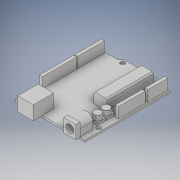
# Autodesk Inventor part: arduinoUno
Saved by Autodesk Inventor 2018 (Build 220112000, 112)
## iProperties
Created: 2020-03-26
Part Number: arduinoUno
Material: Generic
Document SubType Name: Modeling
Designer: natha
Density: 1 g/cm^3
Appearance: Default
Author: natha
Autodesk Inventor part; units mm, degrees
ref_plane "YZ Plane" through (0, 0, 0) normal (1, 0, 0) x (0, 1, 0)
ref_plane "XZ Plane" through (0, 0, 0) normal (0, 1, 0) x (-1, 0, 0)
ref_plane "XY Plane" through (0, 0, 0) normal (0, 0, 1) x (1, 0, 0)
sketch "Sketch1" plane through (0, 0, 0) normal (0, 1, 0) x (-1, 0, 0)
  line L0 (0, 0) -> (53.4, 0)
  line L1 (5, -68.6) -> (2.3639, -65.9639)
  line L2 (5, -68.6) -> (8.728, -68.6) construction
  line L3 (2.3639, -65.9639) -> (0.3639, -65.9639)
  line L4 (0.3639, -65.9639) -> (0, -65.6)
  line L5 (52.7794, -66.2206) -> (53.4, -65.6)
  line L6 (52.7794, -66.2206) -> (40.7794, -66.2206)
  line L7 (40.7794, -66.2206) -> (37.9652, -68.6)
  line L8 (37.9652, -68.6) -> (5, -68.6)
  line L9 (53.4, -65.6) -> (53.4, 0)
  line L10 (0, 0) -> (0, -65.6)
  circle A0 centre (36.6794, -65.9103) radius 1.7
  circle A1 centre (6.3639, -65.6) radius 1.7
  dimension "d2" = 135
  dimension "d3" = 135
  dimension "d10" = 12
  dimension "d12" = 135
  dimension "d13" = 3.4
  dimension "d14" = 3.4
  dimension "d15" = 4.1
  dimension "d16" = 4
  constraints: 22 end point, 5 horizontal, 2 centre point, 1 equal length, 1 perpendicular, 1 vertical
  measures "d2" angle of L2 L1
  measures "d3" angle of L3 L4
  measures "d10" distance of L5.start L6.end
  measures "d12" angle of L6 L5
  measures "d13" diameter of A0
  measures "d14" diameter of A1
  measures "d15" horizontal distance of A0.centre L6.end
  measures "d16" horizontal distance of L1.end A1.centre
extrude "Extrusion1" add sketch "Sketch1" along normal blind 1.5
sketch "Sketch2" plane through (0, 1.5, 0) normal (0, 1, 0) x (1, 0, 0)
  circle A0 centre (-50.9, 14.75) radius 1.7
  line L0 (-53.4, 0) -> (0, 0) projected
  line L1 (-53.4, 65.6) -> (-53.4, 0) projected
  circle A1 centre (-2.5, 13.4) radius 1.7
  line L2 (0, 0) -> (0, 65.6) projected
  dimension "d19" = 3.4
  dimension "d20" = 14.75
  dimension "d21" = 2.5
  dimension "d22" = 3.4
  dimension "d23" = 13.4
  dimension "d24" = 2.5
  constraints: 2 centre point
  measures "d19" diameter of A0
  measures "d20" distance from line of L0 A0.centre
  measures "d21" distance from line of L1 A0.centre
  measures "d22" diameter of A1
  measures "d23" distance from line of L0 A1.centre
  measures "d24" distance from line of L2 A1.centre
extrude "Extrusion2" cut sketch "Sketch2" against normal blind 1.5
sketch "Sketch3" plane through (0, 1.5, 0) normal (0, 1, 0) x (1, 0, 0)
  line L0 (-1, 64.9639) -> (-3.3, 64.9639)
  line L1 (-3.3, 64.9639) -> (-3.3, 49.4639)
  line L2 (-3.3, 49.4639) -> (-1, 49.4639)
  line L3 (-1, 49.4639) -> (-1, 64.9639)
  line L4 (-0.3639, 65.9639) -> (-2.3639, 65.9639) projected
  line L5 (0, 0) -> (0, 65.6) projected
  line L6 (-3.3, 47.4639) -> (-1, 47.4639)
  line L7 (-1, 47.4639) -> (-1, 26.9639)
  line L8 (-1, 26.9639) -> (-3.3, 26.9639)
  line L9 (-3.3, 26.9639) -> (-3.3, 47.4639)
  line L10 (-52.4, 44.7206) -> (-50.1, 44.7206)
  line L11 (-50.1, 44.7206) -> (-50.1, 65.2206)
  line L12 (-50.1, 65.2206) -> (-52.4, 65.2206)
  line L13 (-52.4, 65.2206) -> (-52.4, 44.7206)
  line L14 (-53.4, 65.6) -> (-53.4, 0) projected
  line L15 (-40.7794, 66.2206) -> (-52.7794, 66.2206) projected
  line L16 (-52.4, 43.7206) -> (-50.1, 43.7206)
  line L17 (-50.1, 43.7206) -> (-50.1, 17.6206)
  line L18 (-50.1, 17.6206) -> (-52.4, 17.6206)
  line L19 (-52.4, 17.6206) -> (-52.4, 43.7206)
  dimension "d27" = 1
  dimension "d28" = 15.5
  dimension "d29" = 2.3
  dimension "d30" = 1
  dimension "d31" = 2
  dimension "d32" = 2.3
  dimension "d33" = 20.5
  dimension "d34" = 1
  dimension "d35" = 1
  dimension "d36" = 2.3
  dimension "d37" = 20.5
  dimension "d38" = 26.1
  dimension "d39" = 1
  constraints: 32 end point, 8 parallel, 4 horizontal, 4 perpendicular
  measures "d27" distance between parallel lines of L4 L0
  measures "d28" distance between parallel lines of L2 L0
  measures "d29" distance between parallel lines of L3 L1
  measures "d30" distance between parallel lines of L3 L5
  measures "d31" distance between parallel lines of L2 L6
  measures "d32" distance between parallel lines of L9 L7
  measures "d33" distance between parallel lines of L8 L6
  measures "d34" distance between parallel lines of L14 L13
  measures "d35" distance between parallel lines of L15 L12
  measures "d36" distance between parallel lines of L13 L11
  measures "d37" distance between parallel lines of L10 L12
  measures "d38" distance of L16.end L17.end
  measures "d39" distance between parallel lines of L10 L16
extrude "Extrusion3" add sketch "Sketch3" along normal blind 8.3
sketch "Sketch4" plane through (0, 1.5, 0) normal (0, 1, 0) x (1, 0, 0)
  line L0 (-20.8, 27.85) -> (-10.8, 27.85)
  line L1 (-10.8, 27.85) -> (-10.8, 63.6)
  line L2 (-10.8, 63.6) -> (-20.8, 63.6)
  line L3 (-20.8, 63.6) -> (-20.8, 27.85)
  line L4 (-3.3, 47.4639) -> (-3.3, 26.9639) projected
  line L5 (-5, 68.6) -> (-37.9652, 68.6) projected
  point P0 (0, 0)
  dimension "d42" = 10
  dimension "d43" = 35.75
  dimension "d44" = 7.5
  dimension "d45" = 5
  constraints: 8 end point, 2 parallel, 1 horizontal, 1 perpendicular
  measures "d42" distance of L2.end L1.end
  measures "d43" distance of L1.end L0.end
  measures "d44" distance between parallel lines of L1 L4
  measures "d45" distance between parallel lines of L5 L2
extrude "Extrusion4" add sketch "Sketch4" along normal blind 8
chamfer "Chamfer1" distance 1 angle 45 2 edges at (-20.8, 9.5, -45.725) (-10.8, 9.5, -45.725)
sketch "Sketch5" plane through (0, 1.5, 0) normal (0, 1, 0) x (1, 0, 0)
  line L0 (-4.6091, 14.4286) -> (-11.1091, 14.4286)
  line L1 (-11.1091, 14.4286) -> (-11.1091, 20.9286)
  line L2 (-11.1091, 20.9286) -> (-4.6091, 20.9286)
  line L3 (-4.6091, 20.9286) -> (-4.6091, 14.4286)
  line L4 (-4.6091, 21.1286) -> (-11.1091, 21.1286)
  line L5 (-11.1091, 21.1286) -> (-11.1091, 27.6286)
  line L6 (-11.1091, 27.6286) -> (-4.6091, 27.6286)
  line L7 (-4.6091, 27.6286) -> (-4.6091, 21.1286)
  point P0 (0, 0)
  dimension "d51" = 6.5
  dimension "d52" = 6.5
  dimension "d53" = 6.5
  dimension "d54" = 0.2
  constraints: 16 end point, 4 parallel, 2 horizontal, 2 perpendicular, 2 point on line
  measures "d51" distance of L1.end L2.end
  measures "d52" distance of L0.end L1.end
  measures "d53" distance of L4.end L5.end
  measures "d54" distance between parallel lines of L2 L4
extrude "Extrusion5" add sketch "Sketch5" along normal blind 2
sketch "Sketch6" plane through (0, 3.5, 0) normal (0, 1, 0) x (1, 0, 0)
  circle A0 centre (-7.8591, 17.6786) radius 3
  line L0 (-4.6091, 20.9286) -> (-11.1091, 20.9286) projected
  line L1 (-4.6091, 14.4286) -> (-4.6091, 20.9286) projected
  point P0 (0, 0)
  dimension "d57" = 6
  dimension "d58" = 3.25
  dimension "d59" = 3.25
  constraints: 1 centre point
  measures "d57" diameter of A0
  measures "d58" distance from line of L0 A0.centre
  measures "d59" distance from line of L1 A0.centre
extrude "Extrusion6" add sketch "Sketch6" along normal blind 3.6
sketch "Sketch7" plane through (0, 3.5, 0) normal (0, 1, 0) x (1, 0, 0)
  circle A0 centre (-7.8591, 24.3786) radius 3
  line L0 (-11.1091, 21.1286) -> (-4.6091, 21.1286) projected
  line L1 (-11.1091, 27.6286) -> (-11.1091, 21.1286) projected
  point P0 (0, 0)
  dimension "d62" = 6
  dimension "d63" = 3.25
  dimension "d64" = 3.25
  constraints: 1 centre point
  measures "d62" diameter of A0
  measures "d63" distance from line of L0 A0.centre
  measures "d64" distance from line of L1 A0.centre
extrude "Extrusion7" add sketch "Sketch7" along normal blind 3.6
fillet "Fillet1" radius 0.2 2 edges at (-10.8591, 7.1, -17.6786) (-10.8591, 7.1, -24.3786)
sketch "Sketch8" plane through (0, 1.5, 0) normal (0, 1, 0) x (1, 0, 0)
  line L0 (-52.8, 3) -> (-46.55, 3)
  line L1 (-46.55, 3) -> (-46.55, 9.25)
  line L2 (-46.55, 9.25) -> (-52.8, 9.25)
  line L3 (-52.8, 9.25) -> (-52.8, 3)
  line L4 (-53.4, 65.6) -> (-53.4, 0) projected
  line L5 (-53.4, 0) -> (0, 0) projected
  dimension "d68" = 6.25
  dimension "d69" = 6.25
  dimension "d70" = 0.6
  dimension "d71" = 3
  constraints: 8 end point, 2 parallel, 1 horizontal, 1 perpendicular
  measures "d68" distance of L2.end L1.end
  measures "d69" distance of L1.end L0.end
  measures "d70" distance between parallel lines of L3 L4
  measures "d71" distance between parallel lines of L0 L5
extrude "Extrusion8" add sketch "Sketch8" along normal blind 1.5
sketch "Sketch9" plane through (0, 3, 0) normal (0, 1, 0) x (1, 0, 0)
  circle A0 centre (-49.8, 6) radius 1.5
  line L0 (-46.55, 9.25) -> (-52.8, 9.25) projected
  line L1 (-46.55, 3) -> (-46.55, 9.25) projected
  point P0 (0, 0)
  dimension "d74" = 3
  dimension "d75" = 3.25
  dimension "d76" = 3.25
  constraints: 1 centre point
  measures "d74" diameter of A0
  measures "d75" distance from line of L0 A0.centre
  measures "d76" distance from line of L1 A0.centre
extrude "Extrusion9" add sketch "Sketch9" along normal blind 1
sketch "Sketch10" plane through (0, 1.5, 0) normal (0, 1, 0) x (1, 0, 0)
  line L0 (-12.75, 0) -> (-3.75, 0)
  line L1 (-3.75, 0) -> (-3.75, 10)
  line L2 (-3.75, 10) -> (-12.75, 10)
  line L3 (-12.75, 10) -> (-12.75, 0)
  line L4 (0, 0) -> (0, 65.6) projected
  dimension "d79" = 9
  dimension "d80" = 10
  dimension "d81" = 3.75
  constraints: 8 end point, 2 parallel, 1 horizontal, 1 perpendicular
  measures "d79" distance of L2.end L1.end
  measures "d80" distance of L1.end L0.end
  measures "d81" distance between parallel lines of L4 L1
extrude "Extrusion10" add sketch "Sketch10" along normal blind 10
sketch "Sketch11" plane through (-53.4, 0, 0) normal (0, 0, 1) x (1, 0, 0)
  line L0 (42.6, 1.5) -> (32.6, 1.5) projected
  line L1 (40.5024, 1.5) -> (49.871, 1.5)
  line L2 (49.871, 1.5) -> (49.871, 11.6818)
  line L3 (49.871, 11.6818) -> (40.5024, 11.6818)
  line L4 (40.5024, 11.6818) -> (40.5024, 1.5)
  point P0 (53.4, 0)
  constraints: 8 end point, 2 parallel, 1 horizontal, 1 perpendicular, 1 point on line
extrude "Extrusion11" add sketch "Sketch11" along normal blind 3.2
fillet "Fillet2" radius 4.5 2 edges at (-3.75, 11.5, -5) (-12.75, 11.5, -5)
sketch "Sketch12" plane through (-53.4, 0, 3.2) normal (0, 0, 1) x (1, 0, 0)
  circle A0 centre (45.1865, 6.591) radius 3.125
  line L0 (40.5024, 1.5) -> (49.871, 1.5) projected
  line L1 (49.871, 1.5) -> (49.871, 11.6818) projected
  point P0 (53.4, 0)
  dimension "d87" = 6.25
  dimension "d88" = 5.091
  dimension "d89" = 4.6845
  constraints: 1 centre point
  measures "d87" diameter of A0
  measures "d88" distance from line of L0 A0.centre
  measures "d89" distance from line of L1 A0.centre
extrude "Extrusion12" cut sketch "Sketch12" against normal blind 12
sketch "Sketch13" plane through (0, 1.5, 0) normal (0, 1, 0) x (1, 0, 0)
  line L0 (-44.5774, 0) -> (-32.5774, 0)
  line L1 (-32.5774, 0) -> (-32.5774, 8.75)
  line L2 (-32.5774, 8.75) -> (-44.5774, 8.75)
  line L3 (-44.5774, 8.75) -> (-44.5774, 0)
  point P0 (0, 0)
  dimension "d92" = 12
  dimension "d93" = 8.75
  constraints: 8 end point, 2 parallel, 1 horizontal, 1 perpendicular
  measures "d92" distance of L2.end L1.end
  measures "d93" distance of L1.end L0.end
extrude "Extrusion13" add sketch "Sketch13" along normal blind 10.65
sketch "Sketch14" plane through (-53.4, 0, 0) normal (0, 0, 1) x (1, 0, 0)
  line L0 (8.8226, 1.5) -> (8.8226, 12.15) projected
  line L1 (48.4, 1.5) -> (15.4348, 1.5) projected
  line L2 (8.8226, 12.15) -> (20.8226, 12.15)
  line L3 (20.8226, 12.15) -> (20.8226, 1.5)
  line L4 (20.8226, 1.5) -> (8.8226, 1.5)
  line L5 (8.8226, 1.5) -> (8.8226, 12.15)
  point P0 (53.4, 0)
  constraints: 8 end point, 2 parallel, 1 horizontal, 1 perpendicular, 1 point on line
extrude "Extrusion14" add sketch "Sketch14" along normal blind 7
body "Solid1"
